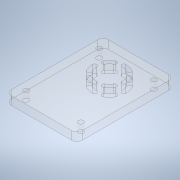
# Autodesk Inventor part: Z_platte_oben_new
Saved by Autodesk Inventor 2022 (Build 260153000, 153)
## iProperties
Created: 2021-04-16
Part Number: Z_platte_oben_new
Material: PET Plastic
Document SubType Name: Modeling
Designer: Fabijan_Sven
Density: 1.541 g/cm^3
Appearance: Polycarbonate - Clear
Mass: 97.0399 g
Surface Area: 201.4 cm^2
Volume: 62.972 cm^3
Author: Fabijan_Sven
Autodesk Inventor part; units mm, degrees
ref_plane "YZ Plane" through (0, 0, 0) normal (1, 0, 0) x (0, 1, 0)
ref_plane "XZ Plane" through (0, 0, 0) normal (0, 1, 0) x (-1, 0, 0)
ref_plane "XY Plane" through (0, 0, 0) normal (0, 0, 1) x (1, 0, 0)
sketch "Sketch1" plane through (0, 0, 0) normal (0, 1, 0) x (-1, 0, 0)
  line L0 (0, 0) -> (68, 0)
  line L1 (68, 0) -> (68, -93)
  line L2 (68, -93) -> (0, -93)
  line L3 (0, -93) -> (0, 0)
  dimension "d0" = 93
  dimension "d1" = 68
  constraints: 8 end point, 2 parallel, 1 horizontal, 1 perpendicular
  measures "d0" distance of L0.end L1.end
  measures "d1" distance of L1.end L2.end
extrude "Extrusion1" add sketch "Sketch1" along normal blind 8
fillet "Fillet1" radius 5 2 edges at (0, 4, -93) (-68, 4, -93)
fillet "Fillet2" radius 5 2 edges at (-68, 4, 0) (0, 4, 0)
sketch "Sketch2" plane through (0, 0, 0) normal (0, -1, 0) x (1, 0, 0)
  circle A0 centre (-7.8137, -81.5) radius 4
  circle A1 centre (-60.1863, -81.5) radius 4
  circle A2 centre (-60.1863, -11.5) radius 4
  circle A3 centre (-7.8137, -11.5) radius 4
  circle A4 centre (-34, -36) radius 4
  point P0 (0, 0)
  dimension "d27" = 70
  dimension "d28" = 52.3726
  dimension "d29" = 8
  dimension "d30" = 24.5
  dimension "d31" = 26.1863
  dimension "d32" = 11.5
  dimension "d33" = 7.8137
  constraints: 5 centre point, 4 equal radius, 2 horizontal alignment, 2 vertical alignment
  measures "d27" distance of A3.centre A0.centre
  measures "d28" distance of A0.centre A1.centre
  measures "d29" diameter of A0
  measures "d30" vertical distance of A3.centre A4.centre
  measures "d31" horizontal distance of A3.centre A4.centre
  measures "d32" vertical distance of point (0, 0) A3.centre
  measures "d33" horizontal distance of point (0, 0) A3.centre
hole "Hole1" at (-7.8137, 0, -81.5) at (-60.1863, 0, -81.5) at (-60.1863, 0, -11.5) at (-7.8137, 0, -11.5) direction (0, 1, 0) diameter 5 end through all
sketch "Sketch3" plane through (0, 8, 0) normal (0, 1, 0) x (1, 0, 0)
  circle A0 centre (-34, 65) radius 11.8188 construction
  line L0 (-63, 0) -> (-5, 0) projected
  line L1 (0, 5) -> (0, 88) projected
  arc A1 (-27, 77.1244) -> (-34, 79) centre (-34, 65) ccw construction
  arc A2 (-26, 78.8564) -> (-34, 81) centre (-34, 65) ccw
  arc A3 (-28, 75.3923) -> (-34, 77) centre (-34, 65) ccw
  arc A4 (-28, 75.3923) -> (-26, 78.8564) centre (-27, 77.1244) ccw
  arc A5 (-34, 81) -> (-34, 77) centre (-34, 79) ccw
  line L2 (-27, 77.1244) -> (-34, 65) construction
  line L3 (-34, 65) -> (-34, 79) construction
  arc A6 (-41, 77.1244) -> (-46.1244, 72) centre (-34, 65) ccw construction
  arc A7 (-42, 78.8564) -> (-47.8564, 73) centre (-34, 65) ccw
  arc A8 (-40, 75.3923) -> (-44.3923, 71) centre (-34, 65) ccw
  arc A9 (-40, 75.3923) -> (-42, 78.8564) centre (-41, 77.1244) ccw
  arc A10 (-47.8564, 73) -> (-44.3923, 71) centre (-46.1244, 72) ccw
  arc A11 (-48, 65) -> (-46.1244, 58) centre (-34, 65) ccw construction
  arc A12 (-50, 65) -> (-47.8564, 57) centre (-34, 65) ccw
  arc A13 (-46, 65) -> (-44.3923, 59) centre (-34, 65) ccw
  arc A14 (-46, 65) -> (-50, 65) centre (-48, 65) ccw
  arc A15 (-47.8564, 57) -> (-44.3923, 59) centre (-46.1244, 58) ccw
  arc A16 (-41, 52.8756) -> (-34, 51) centre (-34, 65) ccw construction
  arc A17 (-42, 51.1436) -> (-34, 49) centre (-34, 65) ccw
  arc A18 (-40, 54.6077) -> (-34, 53) centre (-34, 65) ccw
  arc A19 (-40, 54.6077) -> (-42, 51.1436) centre (-41, 52.8756) ccw
  arc A20 (-34, 49) -> (-34, 53) centre (-34, 51) ccw
  line L4 (-5, 93) -> (-63, 93) projected
  arc A21 (-27, 52.8756) -> (-21.8756, 58) centre (-34, 65) ccw construction
  arc A22 (-26, 51.1436) -> (-20.1436, 57) centre (-34, 65) ccw
  arc A23 (-28, 54.6077) -> (-23.6077, 59) centre (-34, 65) ccw
  arc A24 (-28, 54.6077) -> (-26, 51.1436) centre (-27, 52.8756) ccw
  arc A25 (-20.1436, 57) -> (-23.6077, 59) centre (-21.8756, 58) ccw
  arc A26 (-20, 65) -> (-21.8756, 72) centre (-34, 65) ccw construction
  arc A27 (-18, 65) -> (-20.1436, 73) centre (-34, 65) ccw
  arc A28 (-22, 65) -> (-23.6077, 71) centre (-34, 65) ccw
  arc A29 (-22, 65) -> (-18, 65) centre (-20, 65) ccw
  arc A30 (-20.1436, 73) -> (-23.6077, 71) centre (-21.8756, 72) ccw
  point P0 (0, 0)
  dimension "d15" = 4
  dimension "d16" = 30
  dimension "d18" = 14
  dimension "d19" = 34
  dimension "d22" = 360
  dimension "d26" = 28
  constraints: 60 point on circle, 31 centre point, 4 end point, 4 tangent, 1 coincident, 1 vertical, 73 other
  measures "d15" diameter of A4
  measures "d16" angle of L2 L3
  measures "d18" distance of L2.end L3.end
  measures "d19" distance from line of L1 A0.centre
  measures "d26" distance from line of L4 A0.centre
extrude "Extrusion2" cut sketch "Sketch3" against normal through all
body "Solid1"
